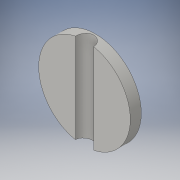
# Autodesk Inventor part: cap
Saved by Autodesk Inventor 2016 (Build 200138000, 138)
## iProperties
Created: 2017-05-30
Part Number: cap
Material: Generic
Document SubType Name: Modeling
Designer: wtse3759
Density: 1 g/cm^3
Appearance: Default
Author: wtse3759
Autodesk Inventor part; units mm, degrees
ref_plane "YZ Plane" through (0, 0, 0) normal (1, 0, 0) x (0, 1, 0)
ref_plane "XZ Plane" through (0, 0, 0) normal (0, 1, 0) x (-1, 0, 0)
ref_plane "XY Plane" through (0, 0, 0) normal (0, 0, 1) x (1, 0, 0)
sketch "Sketch1" plane through (0, 0, 0) normal (0, 0, 1) x (1, 0, 0)
  circle A0 centre (0, 0) radius 6.35
  dimension "d0" = 12.7
  constraints: 1 centre point, 1 coincident
  measures "d0" diameter of A0
extrude "Extrusion1" add sketch "Sketch1" along normal blind 1.524
sketch "Sketch2" plane through (0, 0, 0) normal (0, 1, 0) x (-1, 0, 0)
  line L0 (0, 0) -> (0, 0.254)
  line L1 (6.35, 1.524) -> (-6.35, 1.524) projected
  circle A0 centre (0, 1.524) radius 1.27
  dimension "d3" = 0.254
  constraints: 2 end point, 1 midpoint, 1 vertical, 1 vertical alignment, 2 other
  measures "d3" distance of L0.start L0.end
extrude "Extrusion2" cut sketch "Sketch2" along normal mid plane 12.7
body "Solid1"
